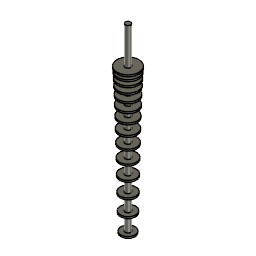
OctoFly(Assemble) (Autodesk Fusion 360 archive; units mm, degrees)
design "OctoLimb"
part number: 2026-05-05-22-04-24-402
Autodesk Fusion 360 part; units mm, degrees
sketch "Sketch1" plane through (0, 0, 0) normal (0, 0, 1) x (1, 0, 0)
  circle A0 centre (0, 0) radius 5
ref_plane "WorkPlane1" through (0, 0, 0) normal (0, 0, 1) x (1, 0, 0)
sketch "Sketch2" plane through (0, 0, 0) normal (0, 0, 1) x (1, 0, 0)
  circle A0 centre (20, 0) radius 1.5
  line L0 (0, -10) -> (0, 10) construction
revolve "Revolve1" add sketch "Sketch2" angle 360 about axis through (0, -10, 0) along (0, 1, 0) makes body 1
ref_plane "WorkPlane2" through (0, 0, 32) normal (0, 0, 1) x (1, 0, 0)
sketch "Sketch3" plane through (0, 0, 32) normal (0, 0, 1) x (1, 0, 0)
  circle A0 centre (19.5, 0) radius 1.5
  line L0 (0, -10) -> (0, 10) construction
revolve "Revolve2" add sketch "Sketch3" angle 360 about axis through (0, -10, 32) along (0, 1, 0) separate body makes body 2
ref_plane "WorkPlane3" through (0, 0, 62) normal (0, 0, 1) x (1, 0, 0)
sketch "Sketch4" plane through (0, 0, 62) normal (0, 0, 1) x (1, 0, 0)
  circle A0 centre (19, 0) radius 1.5
  line L0 (0, -10) -> (0, 10) construction
revolve "Revolve3" add sketch "Sketch4" angle 360 about axis through (0, -10, 62) along (0, 1, 0) separate body makes body 3
ref_plane "WorkPlane4" through (0, 0, 90) normal (0, 0, 1) x (1, 0, 0)
sketch "Sketch5" plane through (0, 0, 90) normal (0, 0, 1) x (1, 0, 0)
  circle A0 centre (18.5, 0) radius 1.5
  line L0 (0, -10) -> (0, 10) construction
revolve "Revolve4" add sketch "Sketch5" angle 360 about axis through (0, -10, 90) along (0, 1, 0) separate body makes body 4
ref_plane "WorkPlane5" through (0, 0, 116) normal (0, 0, 1) x (1, 0, 0)
sketch "Sketch6" plane through (0, 0, 116) normal (0, 0, 1) x (1, 0, 0)
  circle A0 centre (18, 0) radius 1.5
  line L0 (0, -10) -> (0, 10) construction
revolve "Revolve5" add sketch "Sketch6" angle 360 about axis through (0, -10, 116) along (0, 1, 0) separate body makes body 5
ref_plane "WorkPlane6" through (0, 0, 140) normal (0, 0, 1) x (1, 0, 0)
sketch "Sketch7" plane through (0, 0, 140) normal (0, 0, 1) x (1, 0, 0)
  circle A0 centre (17.5, 0) radius 1.5
  line L0 (0, -10) -> (0, 10) construction
revolve "Revolve6" add sketch "Sketch7" angle 360 about axis through (0, -10, 140) along (0, 1, 0) separate body makes body 6
ref_plane "WorkPlane7" through (0, 0, 162) normal (0, 0, 1) x (1, 0, 0)
sketch "Sketch8" plane through (0, 0, 162) normal (0, 0, 1) x (1, 0, 0)
  circle A0 centre (17, 0) radius 1.5
  line L0 (0, -10) -> (0, 10) construction
revolve "Revolve7" add sketch "Sketch8" angle 360 about axis through (0, -10, 162) along (0, 1, 0) separate body makes body 7
ref_plane "WorkPlane8" through (0, 0, 182) normal (0, 0, 1) x (1, 0, 0)
sketch "Sketch9" plane through (0, 0, 182) normal (0, 0, 1) x (1, 0, 0)
  circle A0 centre (16.5, 0) radius 1.5
  line L0 (0, -10) -> (0, 10) construction
revolve "Revolve8" add sketch "Sketch9" angle 360 about axis through (0, -10, 182) along (0, 1, 0) separate body makes body 8
ref_plane "WorkPlane9" through (0, 0, 200) normal (0, 0, 1) x (1, 0, 0)
sketch "Sketch10" plane through (0, 0, 200) normal (0, 0, 1) x (1, 0, 0)
  circle A0 centre (16, 0) radius 1.5
  line L0 (0, -10) -> (0, 10) construction
revolve "Revolve9" add sketch "Sketch10" angle 360 about axis through (0, -10, 200) along (0, 1, 0) separate body makes body 9
ref_plane "WorkPlane10" through (0, 0, 216) normal (0, 0, 1) x (1, 0, 0)
sketch "Sketch11" plane through (0, 0, 216) normal (0, 0, 1) x (1, 0, 0)
  circle A0 centre (15.5, 0) radius 1.5
  line L0 (0, -10) -> (0, 10) construction
revolve "Revolve10" add sketch "Sketch11" angle 360 about axis through (0, -10, 216) along (0, 1, 0) separate body makes body 10
ref_plane "WorkPlane11" through (0, 0, 230) normal (0, 0, 1) x (1, 0, 0)
sketch "Sketch12" plane through (0, 0, 230) normal (0, 0, 1) x (1, 0, 0)
  circle A0 centre (15, 0) radius 1.5
  line L0 (0, -10) -> (0, 10) construction
revolve "Revolve11" add sketch "Sketch12" angle 360 about axis through (0, -10, 230) along (0, 1, 0) separate body makes body 11
ref_plane "WorkPlane12" through (0, 0, 242) normal (0, 0, 1) x (1, 0, 0)
sketch "Sketch13" plane through (0, 0, 242) normal (0, 0, 1) x (1, 0, 0)
  circle A0 centre (14.5, 0) radius 1.5
  line L0 (0, -10) -> (0, 10) construction
revolve "Revolve12" add sketch "Sketch13" angle 360 about axis through (0, -10, 242) along (0, 1, 0) separate body makes body 12
ref_plane "WorkPlane13" through (0, 0, 252) normal (0, 0, 1) x (1, 0, 0)
sketch "Sketch14" plane through (0, 0, 252) normal (0, 0, 1) x (1, 0, 0)
  circle A0 centre (14, 0) radius 1.5
  line L0 (0, -10) -> (0, 10) construction
revolve "Revolve13" add sketch "Sketch14" angle 360 about axis through (0, -10, 252) along (0, 1, 0) separate body makes body 13
ref_plane "WorkPlane14" through (0, 0, 260) normal (0, 0, 1) x (1, 0, 0)
sketch "Sketch15" plane through (0, 0, 260) normal (0, 0, 1) x (1, 0, 0)
  circle A0 centre (13, 0) radius 1.5
  line L0 (0, -10) -> (0, 10) construction
revolve "Revolve14" add sketch "Sketch15" angle 360 about axis through (0, -10, 260) along (0, 1, 0) separate body makes body 14
sketch "Sketch16" plane through (0, 0, 0) normal (0, 0, 1) x (1, 0, 0)
  circle A0 centre (0, 0) radius 5
ref_plane "WorkPlane15" through (0, 0, 0) normal (0, 0, 1) x (1, 0, 0)
sketch "Sketch17" plane through (0, 0, 0) normal (0, 0, 1) x (1, 0, 0)
  circle A0 centre (0, 0) radius 20
  circle A1 centre (0, 0) radius 5.1
ref_plane "WorkPlane16" through (0, 0, 32) normal (0, 0, 1) x (1, 0, 0)
sketch "Sketch18" plane through (0, 0, 32) normal (0, 0, 1) x (1, 0, 0)
  circle A0 centre (0, 0) radius 19.5
  circle A1 centre (0, 0) radius 5.1
ref_plane "WorkPlane17" through (0, 0, 62) normal (0, 0, 1) x (1, 0, 0)
sketch "Sketch19" plane through (0, 0, 62) normal (0, 0, 1) x (1, 0, 0)
  circle A0 centre (0, 0) radius 19
  circle A1 centre (0, 0) radius 5.1
ref_plane "WorkPlane18" through (0, 0, 90) normal (0, 0, 1) x (1, 0, 0)
sketch "Sketch20" plane through (0, 0, 90) normal (0, 0, 1) x (1, 0, 0)
  circle A0 centre (0, 0) radius 18.5
  circle A1 centre (0, 0) radius 5.1
ref_plane "WorkPlane19" through (0, 0, 116) normal (0, 0, 1) x (1, 0, 0)
sketch "Sketch21" plane through (0, 0, 116) normal (0, 0, 1) x (1, 0, 0)
  circle A0 centre (0, 0) radius 18
  circle A1 centre (0, 0) radius 5.1
ref_plane "WorkPlane20" through (0, 0, 140) normal (0, 0, 1) x (1, 0, 0)
sketch "Sketch22" plane through (0, 0, 140) normal (0, 0, 1) x (1, 0, 0)
  circle A0 centre (0, 0) radius 17.5
  circle A1 centre (0, 0) radius 5.1
ref_plane "WorkPlane21" through (0, 0, 162) normal (0, 0, 1) x (1, 0, 0)
sketch "Sketch23" plane through (0, 0, 162) normal (0, 0, 1) x (1, 0, 0)
  circle A0 centre (0, 0) radius 17
  circle A1 centre (0, 0) radius 5.1
ref_plane "WorkPlane22" through (0, 0, 182) normal (0, 0, 1) x (1, 0, 0)
sketch "Sketch24" plane through (0, 0, 182) normal (0, 0, 1) x (1, 0, 0)
  circle A0 centre (0, 0) radius 16.5
  circle A1 centre (0, 0) radius 5.1
ref_plane "WorkPlane23" through (0, 0, 200) normal (0, 0, 1) x (1, 0, 0)
sketch "Sketch25" plane through (0, 0, 200) normal (0, 0, 1) x (1, 0, 0)
  circle A0 centre (0, 0) radius 16
  circle A1 centre (0, 0) radius 5.1
ref_plane "WorkPlane24" through (0, 0, 216) normal (0, 0, 1) x (1, 0, 0)
sketch "Sketch26" plane through (0, 0, 216) normal (0, 0, 1) x (1, 0, 0)
  circle A0 centre (0, 0) radius 15.5
  circle A1 centre (0, 0) radius 5.1
ref_plane "WorkPlane25" through (0, 0, 230) normal (0, 0, 1) x (1, 0, 0)
sketch "Sketch27" plane through (0, 0, 230) normal (0, 0, 1) x (1, 0, 0)
  circle A0 centre (0, 0) radius 15
  circle A1 centre (0, 0) radius 5.1
ref_plane "WorkPlane26" through (0, 0, 242) normal (0, 0, 1) x (1, 0, 0)
sketch "Sketch28" plane through (0, 0, 242) normal (0, 0, 1) x (1, 0, 0)
  circle A0 centre (0, 0) radius 14.5
  circle A1 centre (0, 0) radius 5.1
ref_plane "WorkPlane27" through (0, 0, 252) normal (0, 0, 1) x (1, 0, 0)
sketch "Sketch29" plane through (0, 0, 252) normal (0, 0, 1) x (1, 0, 0)
  circle A0 centre (0, 0) radius 14
  circle A1 centre (0, 0) radius 5.1
ref_plane "WorkPlane28" through (0, 0, 260) normal (0, 0, 1) x (1, 0, 0)
sketch "Sketch30" plane through (0, 0, 260) normal (0, 0, 1) x (1, 0, 0)
  circle A0 centre (0, 0) radius 13
  circle A1 centre (0, 0) radius 5.1
sketch "Sketch31" plane through (0, 0, 0) normal (0, 0, 1) x (1, 0, 0)
  circle A0 centre (0, 0) radius 5
ref_plane "WorkPlane29" through (0, 0, 0) normal (0, 0, 1) x (1, 0, 0)
sketch "Sketch32" plane through (0, 0, 0) normal (0, 0, 1) x (1, 0, 0)
  circle A0 centre (0, 0) radius 13
  circle A1 centre (0, 0) radius 5.1
ref_plane "WorkPlane30" through (0, 0, 32) normal (0, 0, 1) x (1, 0, 0)
sketch "Sketch33" plane through (0, 0, 32) normal (0, 0, 1) x (1, 0, 0)
  circle A0 centre (0, 0) radius 14
  circle A1 centre (0, 0) radius 5.1
ref_plane "WorkPlane31" through (0, 0, 62) normal (0, 0, 1) x (1, 0, 0)
sketch "Sketch34" plane through (0, 0, 62) normal (0, 0, 1) x (1, 0, 0)
  circle A0 centre (0, 0) radius 14.5
  circle A1 centre (0, 0) radius 5.1
ref_plane "WorkPlane32" through (0, 0, 90) normal (0, 0, 1) x (1, 0, 0)
sketch "Sketch35" plane through (0, 0, 90) normal (0, 0, 1) x (1, 0, 0)
  circle A0 centre (0, 0) radius 15
  circle A1 centre (0, 0) radius 5.1
ref_plane "WorkPlane33" through (0, 0, 116) normal (0, 0, 1) x (1, 0, 0)
sketch "Sketch36" plane through (0, 0, 116) normal (0, 0, 1) x (1, 0, 0)
  circle A0 centre (0, 0) radius 15.5
  circle A1 centre (0, 0) radius 5.1
ref_plane "WorkPlane34" through (0, 0, 140) normal (0, 0, 1) x (1, 0, 0)
sketch "Sketch37" plane through (0, 0, 140) normal (0, 0, 1) x (1, 0, 0)
  circle A0 centre (0, 0) radius 16
  circle A1 centre (0, 0) radius 5.1
ref_plane "WorkPlane35" through (0, 0, 162) normal (0, 0, 1) x (1, 0, 0)
sketch "Sketch38" plane through (0, 0, 162) normal (0, 0, 1) x (1, 0, 0)
  circle A0 centre (0, 0) radius 16.5
  circle A1 centre (0, 0) radius 5.1
ref_plane "WorkPlane36" through (0, 0, 182) normal (0, 0, 1) x (1, 0, 0)
sketch "Sketch39" plane through (0, 0, 182) normal (0, 0, 1) x (1, 0, 0)
  circle A0 centre (0, 0) radius 17
  circle A1 centre (0, 0) radius 5.1
ref_plane "WorkPlane37" through (0, 0, 200) normal (0, 0, 1) x (1, 0, 0)
sketch "Sketch40" plane through (0, 0, 200) normal (0, 0, 1) x (1, 0, 0)
  circle A0 centre (0, 0) radius 17.5
  circle A1 centre (0, 0) radius 5.1
ref_plane "WorkPlane38" through (0, 0, 216) normal (0, 0, 1) x (1, 0, 0)
sketch "Sketch41" plane through (0, 0, 216) normal (0, 0, 1) x (1, 0, 0)
  circle A0 centre (0, 0) radius 18
  circle A1 centre (0, 0) radius 5.1
ref_plane "WorkPlane39" through (0, 0, 230) normal (0, 0, 1) x (1, 0, 0)
sketch "Sketch42" plane through (0, 0, 230) normal (0, 0, 1) x (1, 0, 0)
  circle A0 centre (0, 0) radius 18.5
  circle A1 centre (0, 0) radius 5.1
ref_plane "WorkPlane40" through (0, 0, 242) normal (0, 0, 1) x (1, 0, 0)
sketch "Sketch43" plane through (0, 0, 242) normal (0, 0, 1) x (1, 0, 0)
  circle A0 centre (0, 0) radius 19
  circle A1 centre (0, 0) radius 5.1
ref_plane "WorkPlane41" through (0, 0, 252) normal (0, 0, 1) x (1, 0, 0)
sketch "Sketch44" plane through (0, 0, 252) normal (0, 0, 1) x (1, 0, 0)
  circle A0 centre (0, 0) radius 19.5
  circle A1 centre (0, 0) radius 5.1
ref_plane "WorkPlane42" through (0, 0, 260) normal (0, 0, 1) x (1, 0, 0)
sketch "Sketch45" plane through (0, 0, 260) normal (0, 0, 1) x (1, 0, 0)
  circle A0 centre (0, 0) radius 20
  circle A1 centre (0, 0) radius 5.1
sketch "Sketch46" plane through (0, 0, 0) normal (0, 0, 1) x (1, 0, 0)
  circle A0 centre (6, 0) radius 0.5
delete_face "DeleteFace1" 14 faces at (19.5149, -0.513, 8.8055) (2.1026, 0.513, 199.2217) (-6.8095, -0.513, 108.7088) (4.9077, -0.513, 237.3929) (-0.434, 0.513, 182.5959) (-4.5427, -0.513, 179.8403) (5.9265, -0.513, 273.1344) (-9.7609, -0.513, 44.0759) (-10.0001, -0.513, 50.3632) (2.0404, 0.513, 213.7178) (-1.9783, 0.513, 257.7861) (-15.3534, -0.513, 151.0383) (6.1254, -0.513, 198.8295) (-9.2827, 0.513, 133.0459) on bodies 1 2 3 4 5 6 7 8 9 10 11 12 13 14
sketch "Sketch47" plane through (0, 0, 0) normal (0, 0, 1) x (1, 0, 0)
  circle A0 centre (0, 0) radius 5
extrude "Extrude33" add sketch "Sketch47" along normal blind 330.2 separate body makes body 15
ref_plane "WorkPlane43" through (0, 0, 0) normal (0, 0, 1) x (1, 0, 0)
sketch "Sketch48" plane through (0, 0, 0) normal (0, 0, 1) x (1, 0, 0)
  circle A0 centre (0, 0) radius 13
  circle A1 centre (0, 0) radius 5.1
extrude "Extrude34" add sketch "Sketch48" along normal blind 3 separate body makes body 16
ref_plane "WorkPlane44" through (0, 0, 32) normal (0, 0, 1) x (1, 0, 0)
sketch "Sketch49" plane through (0, 0, 32) normal (0, 0, 1) x (1, 0, 0)
  circle A0 centre (0, 0) radius 14
  circle A1 centre (0, 0) radius 5.1
extrude "Extrude35" add sketch "Sketch49" along normal blind 3 separate body makes body 17
ref_plane "WorkPlane45" through (0, 0, 62) normal (0, 0, 1) x (1, 0, 0)
sketch "Sketch50" plane through (0, 0, 62) normal (0, 0, 1) x (1, 0, 0)
  circle A0 centre (0, 0) radius 14.5
  circle A1 centre (0, 0) radius 5.1
extrude "Extrude36" add sketch "Sketch50" along normal blind 3 separate body makes body 18
ref_plane "WorkPlane46" through (0, 0, 90) normal (0, 0, 1) x (1, 0, 0)
sketch "Sketch51" plane through (0, 0, 90) normal (0, 0, 1) x (1, 0, 0)
  circle A0 centre (0, 0) radius 15
  circle A1 centre (0, 0) radius 5.1
extrude "Extrude37" add sketch "Sketch51" along normal blind 3 separate body makes body 19
ref_plane "WorkPlane47" through (0, 0, 116) normal (0, 0, 1) x (1, 0, 0)
sketch "Sketch52" plane through (0, 0, 116) normal (0, 0, 1) x (1, 0, 0)
  circle A0 centre (0, 0) radius 15.5
  circle A1 centre (0, 0) radius 5.1
extrude "Extrude38" add sketch "Sketch52" along normal blind 3 separate body makes body 20
ref_plane "WorkPlane48" through (0, 0, 140) normal (0, 0, 1) x (1, 0, 0)
sketch "Sketch53" plane through (0, 0, 140) normal (0, 0, 1) x (1, 0, 0)
  circle A0 centre (0, 0) radius 16
  circle A1 centre (0, 0) radius 5.1
extrude "Extrude39" add sketch "Sketch53" along normal blind 3 separate body makes body 21
ref_plane "WorkPlane49" through (0, 0, 162) normal (0, 0, 1) x (1, 0, 0)
sketch "Sketch54" plane through (0, 0, 162) normal (0, 0, 1) x (1, 0, 0)
  circle A0 centre (0, 0) radius 16.5
  circle A1 centre (0, 0) radius 5.1
extrude "Extrude40" add sketch "Sketch54" along normal blind 3 separate body makes body 22
ref_plane "WorkPlane50" through (0, 0, 182) normal (0, 0, 1) x (1, 0, 0)
sketch "Sketch55" plane through (0, 0, 182) normal (0, 0, 1) x (1, 0, 0)
  circle A0 centre (0, 0) radius 17
  circle A1 centre (0, 0) radius 5.1
extrude "Extrude41" add sketch "Sketch55" along normal blind 3 separate body makes body 23
ref_plane "WorkPlane51" through (0, 0, 200) normal (0, 0, 1) x (1, 0, 0)
sketch "Sketch56" plane through (0, 0, 200) normal (0, 0, 1) x (1, 0, 0)
  circle A0 centre (0, 0) radius 17.5
  circle A1 centre (0, 0) radius 5.1
extrude "Extrude42" add sketch "Sketch56" along normal blind 3 separate body makes body 24
ref_plane "WorkPlane52" through (0, 0, 216) normal (0, 0, 1) x (1, 0, 0)
sketch "Sketch57" plane through (0, 0, 216) normal (0, 0, 1) x (1, 0, 0)
  circle A0 centre (0, 0) radius 18
  circle A1 centre (0, 0) radius 5.1
extrude "Extrude43" add sketch "Sketch57" along normal blind 3 separate body makes body 25
ref_plane "WorkPlane53" through (0, 0, 230) normal (0, 0, 1) x (1, 0, 0)
sketch "Sketch58" plane through (0, 0, 230) normal (0, 0, 1) x (1, 0, 0)
  circle A0 centre (0, 0) radius 18.5
  circle A1 centre (0, 0) radius 5.1
extrude "Extrude44" add sketch "Sketch58" along normal blind 3 separate body makes body 26
ref_plane "WorkPlane54" through (0, 0, 242) normal (0, 0, 1) x (1, 0, 0)
sketch "Sketch59" plane through (0, 0, 242) normal (0, 0, 1) x (1, 0, 0)
  circle A0 centre (0, 0) radius 19
  circle A1 centre (0, 0) radius 5.1
extrude "Extrude45" add sketch "Sketch59" along normal blind 3 separate body makes body 27
ref_plane "WorkPlane55" through (0, 0, 252) normal (0, 0, 1) x (1, 0, 0)
sketch "Sketch60" plane through (0, 0, 252) normal (0, 0, 1) x (1, 0, 0)
  circle A0 centre (0, 0) radius 19.5
  circle A1 centre (0, 0) radius 5.1
extrude "Extrude46" add sketch "Sketch60" along normal blind 3 separate body makes body 28
ref_plane "WorkPlane56" through (0, 0, 260) normal (0, 0, 1) x (1, 0, 0)
sketch "Sketch61" plane through (0, 0, 260) normal (0, 0, 1) x (1, 0, 0)
  circle A0 centre (0, 0) radius 20
  circle A1 centre (0, 0) radius 5.1
extrude "Extrude47" add sketch "Sketch61" along normal blind 3 separate body makes body 29
sketch "Sketch62" plane through (0, 0, 0) normal (0, 0, 1) x (1, 0, 0)
  circle A0 centre (6, 0) radius 0.5
extrude "Extrude48" add sketch "Sketch62" along normal blind 330.2 separate body makes body 30

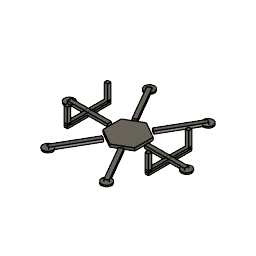
design "HexacopterFrame(OctoFly)"
part number: 2026-05-07-23-01-08-610
Autodesk Fusion 360 part; units mm, degrees
sketch "Sketch1" plane through (0, 0, 0) normal (0, 0, 1) x (1, 0, 0)
  line L0 (47.6314, 27.5) -> (0, 55)
  line L1 (0, 55) -> (-47.6314, 27.5)
  line L2 (-47.6314, 27.5) -> (-47.6314, -27.5)
  line L3 (-47.6314, -27.5) -> (0, -55)
  line L4 (0, -55) -> (47.6314, -27.5)
  line L5 (47.6314, -27.5) -> (47.6314, 27.5)
extrude "Extrude1" add sketch "Sketch1" along normal blind 8 makes body 1
sketch "Sketch2" plane through (0, 0, 0) normal (0, 0, 1) x (1, 0, 0)
  line L0 (55, 6) -> (55, -6)
  line L1 (55, -6) -> (175, -6)
  line L2 (175, -6) -> (175, 6)
  line L3 (175, 6) -> (55, 6)
extrude "Extrude2" add sketch "Sketch2" along normal blind 8 separate body makes body 2
sketch "Sketch3" plane through (0, 0, 0) normal (0, 0, 1) x (1, 0, 0)
  circle A0 centre (175, 0) radius 15
extrude "Extrude3" add sketch "Sketch3" along normal blind 4 separate body makes body 3
sketch "Sketch4" plane through (0, 0, 0) normal (0, 0, 1) x (1, 0, 0)
  line L0 (22.3038, 50.6314) -> (32.6962, 44.6314)
  line L1 (32.6962, 44.6314) -> (92.6962, 148.5544)
  line L2 (92.6962, 148.5544) -> (82.3038, 154.5544)
  line L3 (82.3038, 154.5544) -> (22.3038, 50.6314)
extrude "Extrude4" add sketch "Sketch4" along normal blind 8 separate body makes body 4
sketch "Sketch5" plane through (0, 0, 0) normal (0, 0, 1) x (1, 0, 0)
  circle A0 centre (87.5, 151.5544) radius 15
extrude "Extrude5" add sketch "Sketch5" along normal blind 4 separate body makes body 5
sketch "Sketch6" plane through (0, 0, 0) normal (0, 0, 1) x (1, 0, 0)
  line L0 (-32.6962, 44.6314) -> (-22.3038, 50.6314)
  line L1 (-22.3038, 50.6314) -> (-82.3038, 154.5544)
  line L2 (-82.3038, 154.5544) -> (-92.6962, 148.5544)
  line L3 (-92.6962, 148.5544) -> (-32.6962, 44.6314)
extrude "Extrude6" add sketch "Sketch6" along normal blind 8 separate body makes body 6
sketch "Sketch7" plane through (0, 0, 0) normal (0, 0, 1) x (1, 0, 0)
  circle A0 centre (-87.5, 151.5544) radius 15
extrude "Extrude7" add sketch "Sketch7" along normal blind 4 separate body makes body 7
sketch "Sketch8" plane through (0, 0, 0) normal (0, 0, 1) x (1, 0, 0)
  line L0 (-55, -6) -> (-55, 6)
  line L1 (-55, 6) -> (-175, 6)
  line L2 (-175, 6) -> (-175, -6)
  line L3 (-175, -6) -> (-55, -6)
extrude "Extrude8" add sketch "Sketch8" along normal blind 8 separate body makes body 8
sketch "Sketch9" plane through (0, 0, 0) normal (0, 0, 1) x (1, 0, 0)
  circle A0 centre (-175, 0) radius 15
extrude "Extrude9" add sketch "Sketch9" along normal blind 4 separate body makes body 9
sketch "Sketch10" plane through (0, 0, 0) normal (0, 0, 1) x (1, 0, 0)
  line L0 (-22.3038, -50.6314) -> (-32.6962, -44.6314)
  line L1 (-32.6962, -44.6314) -> (-92.6962, -148.5544)
  line L2 (-92.6962, -148.5544) -> (-82.3038, -154.5544)
  line L3 (-82.3038, -154.5544) -> (-22.3038, -50.6314)
extrude "Extrude10" add sketch "Sketch10" along normal blind 8 separate body makes body 10
sketch "Sketch11" plane through (0, 0, 0) normal (0, 0, 1) x (1, 0, 0)
  circle A0 centre (-87.5, -151.5544) radius 15
extrude "Extrude11" add sketch "Sketch11" along normal blind 4 separate body makes body 11
sketch "Sketch12" plane through (0, 0, 0) normal (0, 0, 1) x (1, 0, 0)
  line L0 (32.6962, -44.6314) -> (22.3038, -50.6314)
  line L1 (22.3038, -50.6314) -> (82.3038, -154.5544)
  line L2 (82.3038, -154.5544) -> (92.6962, -148.5544)
  line L3 (92.6962, -148.5544) -> (32.6962, -44.6314)
extrude "Extrude12" add sketch "Sketch12" along normal blind 8 separate body makes body 12
sketch "Sketch13" plane through (0, 0, 0) normal (0, 0, 1) x (1, 0, 0)
  circle A0 centre (87.5, -151.5544) radius 15
extrude "Extrude13" add sketch "Sketch13" along normal blind 4 separate body makes body 13
sketch "Sketch14" plane through (0, 0, 0) normal (0, 0, 1) x (1, 0, 0)
  line L0 (-126, 55) -> (-116, 55)
  line L1 (-116, 55) -> (-116, 65)
  line L2 (-116, 65) -> (-126, 65)
  line L3 (-126, 65) -> (-126, 55)
extrude "Extrude14" add sketch "Sketch14" along normal blind 50 separate body makes body 14
sketch "Sketch15" plane through (0, 0, 0) normal (0, 0, 1) x (1, 0, 0)
  line L0 (-126, -65) -> (-116, -65)
  line L1 (-116, -65) -> (-116, -55)
  line L2 (-116, -55) -> (-126, -55)
  line L3 (-126, -55) -> (-126, -65)
extrude "Extrude15" add sketch "Sketch15" along normal blind 50 separate body makes body 15
sketch "Sketch16" plane through (0, 0, 0) normal (0, 0, 1) x (1, 0, 0)
  line L0 (-126, -65) -> (-116, -65)
  line L1 (-116, -65) -> (-116, 65)
  line L2 (-116, 65) -> (-126, 65)
  line L3 (-126, 65) -> (-126, -65)
extrude "Extrude16" add sketch "Sketch16" along normal mid plane 12 separate body makes body 16
sketch "Sketch17" plane through (0, 0, 0) normal (0, 0, 1) x (1, 0, 0)
  line L0 (-126, -60) -> (-116, -60)
  line L1 (-116, -60) -> (-116, 60)
  line L2 (-116, 60) -> (-126, 60)
  line L3 (-126, 60) -> (-126, -60)
extrude "Extrude17" add sketch "Sketch17" along normal blind 6 separate body makes body 17
sketch "Sketch18" plane through (0, 0, 0) normal (0, 0, 1) x (1, 0, 0)
  line L0 (116, 55) -> (126, 55)
  line L1 (126, 55) -> (126, 65)
  line L2 (126, 65) -> (116, 65)
  line L3 (116, 65) -> (116, 55)
extrude "Extrude18" add sketch "Sketch18" along normal blind 50 separate body makes body 18
sketch "Sketch19" plane through (0, 0, 0) normal (0, 0, 1) x (1, 0, 0)
  line L0 (116, -65) -> (126, -65)
  line L1 (126, -65) -> (126, -55)
  line L2 (126, -55) -> (116, -55)
  line L3 (116, -55) -> (116, -65)
extrude "Extrude19" add sketch "Sketch19" along normal blind 50 separate body makes body 19
sketch "Sketch20" plane through (0, 0, 0) normal (0, 0, 1) x (1, 0, 0)
  line L0 (116, -65) -> (126, -65)
  line L1 (126, -65) -> (126, 65)
  line L2 (126, 65) -> (116, 65)
  line L3 (116, 65) -> (116, -65)
extrude "Extrude20" add sketch "Sketch20" along normal mid plane 12 separate body makes body 20
sketch "Sketch21" plane through (0, 0, 0) normal (0, 0, 1) x (1, 0, 0)
  line L0 (116, -60) -> (126, -60)
  line L1 (126, -60) -> (126, 60)
  line L2 (126, 60) -> (116, 60)
  line L3 (116, 60) -> (116, -60)
extrude "Extrude21" add sketch "Sketch21" along normal blind 6 separate body makes body 21
